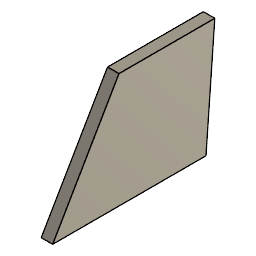
Oct20_Fin (Autodesk Fusion 360 design; units mm, degrees)
part number: 2025-10-20-22-41-00-755
Autodesk Fusion 360 part; units mm, degrees
sketch "Sketch1" plane through (0, 0, 0) normal (1, 0, 0) x (0, 1, 0)
  line L0 (0, 0) -> (40, 0)
  line L1 (40, 0) -> (42.3, 29.9117)
  line L2 (42.3, 29.9117) -> (17.3, 29.9117)
  line L3 (17.3, 29.9117) -> (0, 0)
  dimension "d1" = 40
  dimension "d3" = 25
  dimension "d4" = 30
  constraint coincident L0.start L3.end
  constraint horizontal L0
  constraint parallel L0 L2
  measures "d1" distance of L0.start L0.end
  measures "d3" distance of L1.end L2.end
  measures "d4" distance of L0.end L1.end
extrude "Extrude1" add sketch "Sketch1" along normal blind 3
